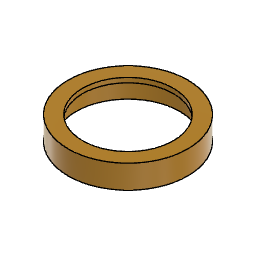
Dichtungsring Einhell Absaugadapter v9 (Autodesk Fusion 360 design; units mm, degrees)
Autodesk Fusion 360 part; units mm, degrees
note: some values were not read from the file. Set by a fixed rule: which sketch regions a step uses.
sketch "Skizze1" plane through (0, 0, 0) normal (1, 0, 0) x (0, 1, 0)
  line L0 (0, 0) -> (19.8, 0) construction
  line L1 (22.2, -2) -> (22.2, -8)
  line L2 (25.5, -8) -> (25.5, 0)
  line L3 (25.5, 0) -> (20.2, 0)
  line L4 (0, 0) -> (23.4577, 0) construction
  line L5 (0, 0) -> (20, 0) construction
  line L6 (19.7, 0) -> (20.2, 0)
  line L7 (22.2, -2) -> (19.4, -2)
  line L8 (19.4, -2) -> (19.3983, 0)
  line L9 (19.3983, 0) -> (20.2, 0)
  line L10 (22.2, -8) -> (22.2, -10)
  line L11 (25.5, -8) -> (25.5, -10)
  line L12 (25.5, -10) -> (22.2, -10)
  point P0 (19.7, 0)
  dimension "d15" = 6
  dimension "d19" = 20
  dimension "d22" = 0.5
  dimension "d24" = 2.8
  dimension "d25" = 0.8017
  constraint coincident L0.start L4.start
  constraint horizontal L0
  constraint coincident L3 L4.end
  constraint parallel L3 L4
  constraint coincident L4 L5.end
  constraint parallel L4 L5
  constraint coincident L3 P0
  constraint coincident L0.end L3
  constraint coincident P0 L6.start
  constraint perpendicular L1 L7
  constraint coincident L5 L8.end
  constraint parallel L6 L9
  constraint parallel L1 L10
  constraint parallel L2 L11
  measures "d15" distance of L1.start L1.end
  measures "d19" distance of L0.start L5.end
  measures "d22" distance of L3.end P0
  measures "d24" distance of L1.start L7.end
  measures "d25" distance of L8.end L3.end
revolve "Drehen1" add sketch "Skizze1" angle 360 about axis through (0, 0, 1.75) along (0, 0, 1)
chamfer "Fase2" [no effect]
